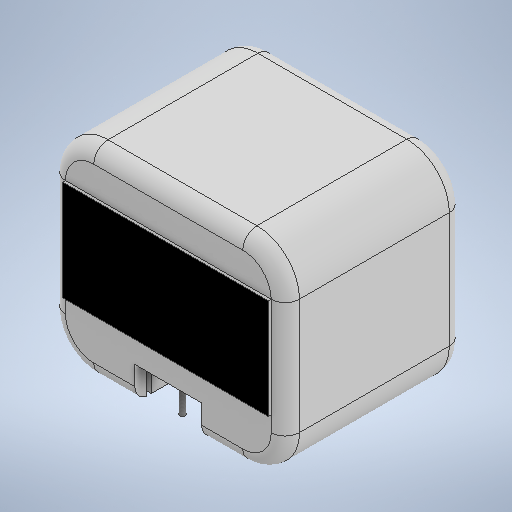
# Autodesk Inventor part: Robot_face
Saved by Autodesk Inventor 2025 (Build 290162010, 162A)
## iProperties
Created: 2024-07-17
Part Number: Robot_face
Material: Generic
Document SubType Name: Modeling
Designer: saees
Density: 1 g/cm^3
Appearance: Default
Author: saees
Autodesk Inventor part; units mm, degrees
ref_plane "YZ Plane" through (0, 0, 0) normal (1, 0, 0) x (0, 1, 0)
ref_plane "XZ Plane" through (0, 0, 0) normal (0, 1, 0) x (-1, 0, 0)
ref_plane "XY Plane" through (0, 0, 0) normal (0, 0, 1) x (1, 0, 0)
sketch "Sketch1" plane through (0, 0, 0) normal (0, 0, 1) x (1, 0, 0)
  line L0 (100.9409, 69.2591) -> (234.7409, 69.2591)
  line L1 (272.8409, 107.3591) -> (272.8409, 211.1591)
  line L2 (234.7409, 249.2591) -> (100.9409, 249.2591)
  line L3 (62.8409, 211.1591) -> (62.8409, 107.3591)
  arc A0 (100.9409, 249.2591) -> (62.8409, 211.1591) centre (100.9409, 211.1591) ccw
  arc A1 (272.8409, 211.1591) -> (234.7409, 249.2591) centre (234.7409, 211.1591) ccw
  arc A2 (234.7409, 69.2591) -> (272.8409, 107.3591) centre (234.7409, 107.3591) ccw
  arc A3 (62.8409, 107.3591) -> (100.9409, 69.2591) centre (100.9409, 107.3591) ccw
  point P0 (0, 0)
  point P1 (62.8409, 69.2591)
  point P2 (272.8409, 249.2591)
  point P3 (272.8409, 69.2591)
  dimension "d0" = 210
  dimension "d1" = 180
  dimension "d2" = 38.1
  dimension "d3" = 38.1
  constraints: 8 end point, 8 point on circle, 8 tangent, 6 point on line, 4 centre point, 2 equal radius, 2 parallel, 1 horizontal, 1 perpendicular
  measures "d0" distance of point (62.841, 69.259) point (272.841, 69.259)
  measures "d1" distance of point (272.841, 69.259) point (272.841, 249.259)
  measures "d2" radius of A0
  measures "d3" radius of A1
extrude "Extrusion1" add sketch "Sketch1" along normal blind 160
fillet "Fillet1" radius 12.7 16 edges at (261.6817, 238.0999, 0) (167.8409, 249.2591, 0) (74.0001, 238.0999, 0) (62.8409, 159.2591, 0) (74.0001, 80.4183, 0) (167.8409, 69.2591, 0) (261.6817, 80.4183, 0) (272.8409, 159.2591, 0) (261.6817, 238.0999, 160) (167.8409, 249.2591, 160) (74.0001, 238.0999, 160) (62.8409, 159.2591, 160) (74.0001, 80.4183, 160) (167.8409, 69.2591, 160) (261.6817, 80.4183, 160) (272.8409, 159.2591, 160)
sketch "Sketch2" plane through (0, 0, 160) normal (0, 0, 1) x (1, 0, 0)
  line L0 (234.7409, 69.2591) -> (100.9409, 69.2591) projected
  line L1 (137.8409, 99.2591) -> (197.8409, 99.2591)
  line L2 (197.8409, 99.2591) -> (197.8409, 69.2591)
  line L3 (197.8409, 69.2591) -> (137.8409, 69.2591)
  line L4 (137.8409, 69.2591) -> (137.8409, 99.2591)
  line L5 (234.7409, 81.9591) -> (100.9409, 81.9591) projected
  point P0 (0, 0)
  point P1 (167.8409, 99.2591)
  point P2 (167.8409, 81.9591)
  dimension "d7" = 60
  dimension "d8" = 30
  constraints: 8 end point, 2 midpoint, 2 parallel, 1 horizontal, 1 perpendicular, 1 point on line, 1 vertical alignment
  measures "d7" distance of L1.start L1.end
  measures "d8" distance of L1.end L2.end
extrude "Extrusion2" cut sketch "Sketch2" against normal blind 30
sketch "Sketch3" plane through (137.8409, 99.2591, 160) normal (0, -1, 0) x (1, 0, 0)
  line L0 (96.9, -12.7) -> (-36.9, -12.7) projected
  circle A0 centre (30, -12.7) radius 2.5
  point P0 (-137.8409, -160)
  dimension "d11" = 5
  constraints: 1 centre point, 1 midpoint
  measures "d11" diameter of A0
extrude "Extrusion3" add sketch "Sketch3" along normal blind 30
thread "Thread1" size "12-24 UNC" class "2A" standard "ANSI Unified Screw Threads" full length
sketch "Sketch4" plane through (0, 0, 160) normal (0, 0, 1) x (1, 0, 0)
  line L0 (260.1409, 107.3591) -> (260.1409, 211.1591) projected
  line L1 (75.5409, 211.1591) -> (260.1409, 211.1591)
  line L2 (260.1409, 211.1591) -> (260.1409, 121.1591)
  line L3 (260.1409, 121.1591) -> (75.5409, 121.1591)
  line L4 (75.5409, 121.1591) -> (75.5409, 211.1591)
  point P0 (0, 0)
  dimension "d16" = 90
  constraints: 8 end point, 2 parallel, 1 coincident, 1 horizontal, 1 perpendicular, 1 point on line
  measures "d16" distance of L3.end L1.start
extrude "Extrusion4" add sketch "Sketch4" along normal blind 2.5
sketch "Sketch5" plane through (100.9409, 69.2591, 12.7) normal (0, -1, 0) x (1, 0, 0)
  line L0 (36.9, 134.6) -> (36.9, 147.3) projected
  line L1 (36.9, 147.3) -> (0, 147.3) projected
  line L2 (0, 134.6) -> (0, 147.3) projected
  line L3 (0, 134.6) -> (36.9, 134.6) projected
  line L4 (96.9, 147.3) -> (96.9, 134.6) projected
  line L5 (96.9, 134.6) -> (133.8, 134.6) projected
  line L6 (133.8, 134.6) -> (133.8, 147.3) projected
  line L7 (133.8, 147.3) -> (96.9, 147.3) projected
  line L8 (96.9, 134.6) -> (96.9, 117.3) projected
  line L9 (96.9, 117.3) -> (36.9, 117.3) projected
  line L10 (36.9, 117.3) -> (36.9, 134.6) projected
  line L11 (0, 134.6) -> (36.9, 134.6) projected
  line L12 (0, 0) -> (0, 134.6) projected
  line L13 (133.8, 0) -> (0, 0) projected
  line L14 (133.8, 0) -> (133.8, 134.6) projected
  line L15 (96.9, 134.6) -> (133.8, 134.6) projected
  line L16 (31.9, 136.6) -> (36.9, 136.6)
  line L17 (36.9, 136.6) -> (36.9, 132.6)
  line L18 (36.9, 132.6) -> (31.9, 132.6)
  line L19 (31.9, 132.6) -> (31.9, 136.6)
  line L20 (96.9, 136.6) -> (101.9, 136.6)
  line L21 (101.9, 136.6) -> (101.9, 132.6)
  line L22 (101.9, 132.6) -> (96.9, 132.6)
  line L23 (96.9, 132.6) -> (96.9, 136.6)
  point P0 (-100.9409, -12.7)
  dimension "d19" = 4
  dimension "d20" = 5
  constraints: 16 end point, 4 parallel, 4 point on line, 2 horizontal, 2 perpendicular, 1 collinear, 1 midpoint
  measures "d19" distance of L18.end L16.start
  measures "d20" distance of L16.start L16.end
extrude "Extrusion5" cut sketch "Sketch5" against normal blind 30 contours L3 L19 L16 L0 | L10 L18 L19 L3 | L8 L5 L21 L22 | L4 L20 L21 L5
body "Solid1"
